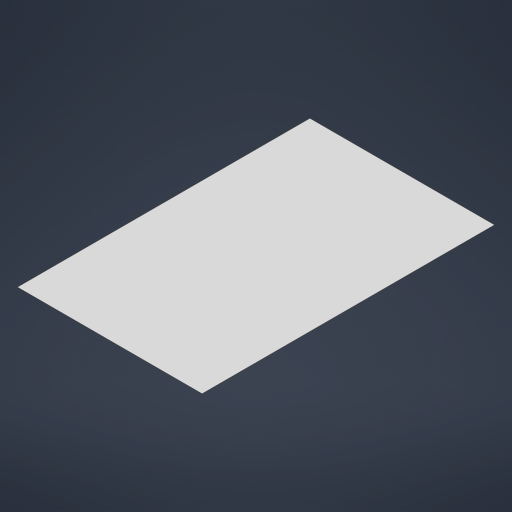
# Autodesk Inventor part: Paper piece
Saved by Autodesk Inventor 2024 (Build 280153000, 153)
## iProperties
Created: 2025-02-12
Part Number: Paper piece
Material: Generic
Document SubType Name: Modeling
Designer: Vincent Larson
Density: 1 g/cm^3
Appearance: Default
Author: Vincent Larson
Autodesk Inventor part; units mm, degrees
ref_plane "YZ Plane" through (0, 0, 0) normal (1, 0, 0) x (0, 1, 0)
ref_plane "XZ Plane" through (0, 0, 0) normal (0, 1, 0) x (-1, 0, 0)
ref_plane "XY Plane" through (0, 0, 0) normal (0, 0, 1) x (1, 0, 0)
sketch "Sketch1" plane through (0, 0, 0) normal (0, 1, 0) x (-1, 0, 0)
  line L0 (-30, 47.5) -> (30, 47.5)
  line L1 (30, 47.5) -> (30, -47.5)
  line L2 (30, -47.5) -> (-30, -47.5)
  line L3 (-30, -47.5) -> (-30, 47.5)
  line L4 (-30, 47.5) -> (30, -47.5) construction
  line L5 (30, 47.5) -> (-30, -47.5) construction
  point P0 (0, 0)
  dimension "d0" = 60
  dimension "d1" = 95
  constraints: 12 end point, 2 midpoint, 2 parallel, 1 horizontal, 1 perpendicular
  measures "d0" distance of L1.end L2.end
  measures "d1" distance of L0.end L1.end
extrude "Extrusion1" add sketch "Sketch1" along normal blind 0.0254
body "Solid1"
